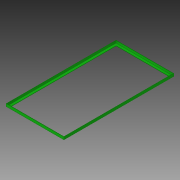
# Autodesk Inventor part: frame
Saved by Autodesk Inventor 2019 (Build 230136000, 136)
## iProperties
Created: 2018-09-24
Part Number: frame
Material: Steel, Mild
Document SubType Name: Modeling
Designer: Callum Snowden
Mass: 3726.47 g
Surface Area: 3360.84 cm^2
Volume: 474.71 cm^3
Density: 7.85 g/cm^3
Appearance: Dark Green
Author: Callum Snowden
Autodesk Inventor part; units mm, degrees
ref_plane "YZ Plane" through (0, 0, 0) normal (1, 0, 0) x (0, 1, 0)
ref_plane "XZ Plane" through (0, 0, 0) normal (0, 1, 0) x (-1, 0, 0)
ref_plane "XY Plane" through (0, 0, 0) normal (0, 0, 1) x (1, 0, 0)
sketch "Sketch1" plane through (0, 0, 0) normal (0, 1, 0) x (-1, 0, 0)
  line L0 (-406, 0) -> (406, 0) construction
  line L1 (0, -773.5) -> (0, 773.5) construction
  line L2 (290, 552.5) -> (-290, 552.5)
  line L3 (-290, 552.5) -> (-290, -552.5)
  line L4 (-290, -552.5) -> (290, -552.5)
  line L5 (290, -552.5) -> (290, 552.5)
  line L6 (264.6, -527.1) -> (-264.6, -527.1)
  line L7 (-264.6, -527.1) -> (-264.6, 527.1)
  line L8 (-264.6, 527.1) -> (264.6, 527.1)
  line L9 (264.6, 527.1) -> (264.6, -527.1)
  point P0 (0, 0)
  dimension "d0" = 580
  dimension "d1" = 1105
  dimension "d8" = 25.4
  dimension "d9" = 25.4
  constraints: 16 end point, 4 parallel, 2 horizontal, 2 perpendicular, 4 other
  measures "d0" distance of L4.end L3.end
  measures "d1" distance of L3.end L2.end
  measures "d8" distance between parallel lines of L5 L9
  measures "d9" distance between parallel lines of L4 L6
extrude "Base thickness" add sketch "Sketch1" along normal blind 3
sketch "Sketch3" plane through (0, 3, 0) normal (0, 1, 0) x (1, 0, 0)
  line L0 (-290, 552.5) -> (-290, -552.5) projected
  line L1 (-290, -552.5) -> (290, -552.5) projected
  line L2 (290, -552.5) -> (290, 552.5) projected
  line L3 (290, 552.5) -> (-290, 552.5) projected
  line L4 (-290, 552.5) -> (-290, -552.5) projected
  line L5 (-287, 549.5) -> (287, 549.5)
  line L6 (287, 549.5) -> (287, -549.5)
  line L7 (287, -549.5) -> (-287, -549.5)
  line L8 (-287, -549.5) -> (-287, 549.5)
  line L9 (0, 773.5) -> (0, -773.5) construction
  line L10 (406, 0) -> (-406, 0) construction
  point P0 (0, 0)
  dimension "d14" = 3
  dimension "d15" = 3
  constraints: 8 end point, 2 parallel, 1 horizontal, 1 perpendicular, 2 other
  measures "d14" distance between parallel lines of L0 L8
  measures "d15" distance between parallel lines of L5 L3
extrude "Wall height" add sketch "Sketch3" along normal blind 22.4
equation "\"d8\" = angleSectionSize"
equation "\"d9\" = angleSectionSize"
equation "\"d12\" = wallThickness"
equation "\"d14\" = wallThickness"
equation "\"d15\" = wallThickness"
equation "\"d16\" = angleSectionSize - wallThickness"
equation "\"wallThickness\" = 3"
equation "\"angleSectionSize\" = 25.4"
body "Solid2"
